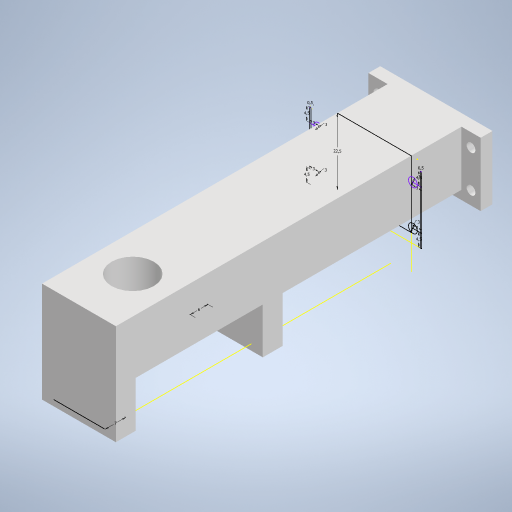
# Autodesk Inventor part: ramie_1
Saved by Autodesk Inventor 2023 (Build 270158000, 158)
## iProperties
Created: 2022-09-14
Part Number: ramie_1
Material: Generic
Document SubType Name: Modeling
Designer: Kamil
Density: 1 g/cm^3
Appearance: Default
Author: Kamil
Autodesk Inventor part; units mm, degrees
ref_plane "YZ Plane" through (0, 0, 0) normal (1, 0, 0) x (0, 1, 0)
ref_plane "XZ Plane" through (0, 0, 0) normal (0, 1, 0) x (-1, 0, 0)
ref_plane "XY Plane" through (0, 0, 0) normal (0, 0, 1) x (1, 0, 0)
sketch "Sketch14" plane through (0, 0, 0) normal (0, 0, 1) x (1, 0, 0)
  line L0 (0, 0) -> (17, 0)
  line L1 (17, 0) -> (17, 30)
  line L2 (17, 30) -> (0, 30)
  line L3 (0, 30) -> (0, 0)
  line L4 (-6, 36) -> (23, 36)
  line L5 (23, 36) -> (23, -6)
  line L6 (23, -6) -> (-6, -6)
  line L7 (-6, -6) -> (-6, 36)
  dimension "d55" = 17
  dimension "d56" = 30
  dimension "d57" = 6
  constraints: 16 end point, 4 parallel, 2 perpendicular, 1 horizontal, 3 other
  measures "d55" distance of L2.end L1.end
  measures "d56" distance of L1.end L0.end
  measures "d57" distance between parallel lines of L2 L4
extrude "Extrusion12" add sketch "Sketch14" against normal blind 3 contours L3 L2 L1 L0 | L4 L5 L6 L7
extrude "Extrusion13" add sketch "Sketch14" along normal blind 90 contours L3 L2 L1 L0
sketch "Sketch15" plane through (0, 0, 0) normal (0, -1, 0) x (1, 0, 0)
  line L0 (0, 0) -> (0, 90) projected
  line L1 (0, 90) -> (17.1111, 90)
  line L2 (0, 90) -> (17, 90)
  line L3 (17, 90) -> (17, 97)
  line L4 (17, 97) -> (0, 97)
  line L5 (0, 97) -> (0, 90)
  line L6 (17, 90) -> (0, 90) projected
  circle A0 centre (3.5, 93.5) radius 1.25
  circle A1 centre (13.5, 93.5) radius 1.25
  line L7 (8.5, 113.1) -> (8.5, 78.8)
  circle A2 centre (8.5, 78.8) radius 7.15
  circle A3 centre (3.5, 44) radius 1.25
  circle A4 centre (13.5, 44) radius 1.25
  line L8 (17, 0) -> (17, 90) projected
  line L9 (0, 97) -> (17, 97)
  line L10 (17, 97) -> (17, 42)
  line L11 (17, 42) -> (0, 42)
  line L12 (0, 42) -> (0, 97)
  line L13 (8.5, 113.1) -> (8.5, 98.4)
  line L14 (3.5, 44) -> (13.5, 44)
  dimension "d67" = 7
  dimension "d70" = 2.5
  dimension "d71" = 2.5
  dimension "d72" = 34.3
  dimension "d73" = 14.3
  dimension "d79" = 55
  dimension "d95" = 14.7
  constraints: 24 end point, 5 centre point, 4 parallel, 3 horizontal, 2 perpendicular, 2 point on line, 1 coincident, 1 vertical
  measures "d67" distance of L3.end L2.end
  measures "d70" diameter of A0
  measures "d71" diameter of A1
  measures "d72" distance of L7.start L7.end
  measures "d73" diameter of A2
  measures "d79" distance of L9.end L10.end
  measures "d95" distance of L7.start L13.end
extrude "Extrusion14" cut sketch "Sketch15" against normal blind 169.375 contours A2
extrude "Extrusion15" cut sketch "Sketch15" against normal blind 15.5 contours L0 L1 L8 L11
extrude "Extrusion16" cut sketch "Sketch15" against normal blind 20 contours A3 | A4
extrude "Extrusion17" add sketch "Sketch15" against normal blind 30 contours L5 L4 L7 L1 | L7 L4 L3 L1
sketch "Sketch16" plane through (0, 0, 0) normal (0, -1, 0) x (1, 0, 0)
  line L0 (0, 0) -> (0, 97) projected
  line L1 (17, 0) -> (17, 97) projected
  line L2 (0, 97) -> (17, 97)
  line L3 (17, 97) -> (17, 90)
  line L4 (17, 90) -> (0, 90)
  line L5 (0, 90) -> (0, 97)
  dimension "d86" = 7
  constraints: 8 end point, 2 parallel, 1 horizontal, 1 perpendicular, 1 point on line
  measures "d86" distance of L2.end L3.end
extrude "Extrusion18" cut sketch "Sketch15" against normal blind 15.5 contours L5 L4 L7 L1 | L7 L4 L3 L1
sketch "Sketch17" plane through (0, 15.5, 0) normal (0, -1, 0) x (1, 0, 0)
  line L0 (0, 97) -> (17, 97) projected
  line L1 (17, 0) -> (17, 97) projected
  line L2 (0, 97) -> (17, 97)
  line L3 (17, 97) -> (17, 91)
  line L4 (17, 91) -> (0, 91)
  line L5 (0, 91) -> (0, 97)
  line L6 (17, 42) -> (0, 42) projected
  line L7 (0, 42) -> (17, 42)
  line L8 (17, 42) -> (17, 47)
  line L9 (17, 47) -> (0, 47)
  line L10 (0, 47) -> (0, 42)
  circle A0 centre (3.5, 44) radius 1.25 projected
  circle A1 centre (3.5, 44) radius 1.25
  circle A2 centre (13.5, 44) radius 1.25 projected
  circle A3 centre (13.5, 44) radius 1.25
  circle A4 centre (3.5, 93.5) radius 1.25 projected
  circle A5 centre (3.5, 93.5) radius 1.25
  circle A6 centre (13.5, 93.5) radius 1.25 projected
  circle A7 centre (13.5, 93.5) radius 1.25
  point P0 (0, 0)
  dimension "d89" = 6
  dimension "d90" = 5
  dimension "d91" = 2.5
  dimension "d92" = 2.5
  constraints: 16 end point, 4 centre point, 4 coincident, 4 parallel, 2 horizontal, 2 perpendicular, 2 point on line
  measures "d89" distance of L2.end L3.end
  measures "d90" distance of L8.end L7.end
  measures "d91" diameter of A5
  measures "d92" diameter of A7
extrude "Extrusion19" add sketch "Sketch17" along normal blind 15.5
sketch "Sketch19" plane through (0, 0, 0) normal (0, -1, 0) x (1, 0, 0)
  line L0 (0, 0) -> (0, 47) projected
  line L1 (17, 0) -> (17, 47) projected
  line L2 (0, 0) -> (17, 0)
  line L3 (17, 0) -> (17, 40)
  line L4 (17, 40) -> (0, 40)
  line L5 (0, 40) -> (0, 0)
  dimension "d96" = 40
  constraints: 8 end point, 2 parallel, 1 horizontal, 1 perpendicular, 1 point on line
  measures "d96" distance of L3.end L2.end
extrude "Extrusion20" cut sketch "Sketch19" against normal blind 15.5
sketch "Sketch23" plane through (0, 0, 0) normal (0, 0, 1) x (1, 0, 0)
  line L0 (0, 15.5) -> (17, 15.5) projected
  line L1 (0, 15.5) -> (0, 9.5)
  line L2 (0, 15.5) -> (0, 0) projected
  line L3 (0, 9.5) -> (-6, 9.5)
  line L4 (-6, -6) -> (-6, 36) projected
  line L5 (23, 36) -> (23, -6) projected
  line L6 (23, 9.5) -> (0, 9.5)
  line L7 (-6, 9.5) -> (23, 9.5)
  line L8 (23, 9.5) -> (23, 36)
  line L9 (23, 36) -> (-6, 36)
  line L10 (-6, 36) -> (-6, 9.5)
  line L11 (23, -6) -> (-6, -6) projected
  line L12 (-6, -6) -> (23, -6)
  line L13 (23, -6) -> (23, 9.5)
  line L14 (23, 9.5) -> (-6, 9.5)
  line L15 (-6, 9.5) -> (-6, -6)
  dimension "d99" = 6
  constraints: 22 end point, 4 parallel, 4 perpendicular, 4 point on line, 2 horizontal
  measures "d99" distance of L0.start L1.end
extrude "Extrusion21" cut sketch "Sketch23" against normal blind 15.5 contours L6 L5 L11 L4 L3
sketch "Sketch24" plane through (0, 30, 97) normal (0, 0, 1) x (1, 0, 0)
  line L0 (17, 0) -> (17, -14.5) projected
  line L1 (17, 0) -> (19, 0)
  line L2 (19, 0) -> (19, 2)
  line L3 (0, -14.5) -> (0, -30) projected
  line L4 (0, -14.5) -> (-2, -14.5)
  line L5 (-2, -14.5) -> (-2, -16.5)
  line L6 (-2, -16.5) -> (19, -16.5)
  line L7 (19, -16.5) -> (19, 2)
  line L8 (19, 2) -> (-2, 2)
  line L9 (-2, 2) -> (-2, -16.5)
  dimension "d111" = 2
  dimension "d112" = 2
  dimension "d113" = 2
  dimension "d114" = 2
  constraints: 16 end point, 3 horizontal, 3 perpendicular, 2 parallel
  measures "d111" distance of L0.start L1.end
  measures "d112" distance of L1.end L2.end
  measures "d113" distance of L3.start L4.end
  measures "d114" distance of L4.end L5.end
extrude "Extrusion22" add sketch "Sketch24" against normal blind 97
extrude "Extrusion23" cut sketch "Sketch15" against normal blind 169.375 contours A2
sketch "Sketch26" plane through (-2, 13.5, 0) normal (0, -1, 0) x (1, 0, 0)
  line L0 (0, 97) -> (2, 97) projected
  line L1 (2, 97) -> (2, 91) projected
  line L2 (0, 97) -> (2, 97)
  line L3 (2, 97) -> (2, 91)
  line L4 (2, 91) -> (0, 91)
  line L5 (0, 91) -> (0, 97)
  line L6 (2, 91) -> (19, 91) projected
  line L7 (19, 97) -> (21, 97) projected
  line L8 (19, 91) -> (21, 91)
  line L9 (21, 91) -> (21, 97)
  line L10 (21, 97) -> (19, 97)
  line L11 (19, 97) -> (19, 91)
  line L12 (2, 40) -> (19, 40) projected
  line L13 (0, 97) -> (0, 0) projected
  line L14 (2, 40) -> (0, 40)
  line L15 (0, 40) -> (0, 47)
  line L16 (0, 47) -> (2, 47)
  line L17 (2, 47) -> (2, 40)
  line L18 (19, 40) -> (19, 47) projected
  line L19 (21, 97) -> (21, 0) projected
  line L20 (19, 40) -> (21, 40)
  line L21 (21, 40) -> (21, 47)
  line L22 (21, 47) -> (19, 47)
  line L23 (19, 47) -> (19, 40)
  point P0 (2, 0)
  point P1 (0, 40)
  dimension "d119" = 7
  constraints: 32 end point, 8 parallel, 4 horizontal, 4 perpendicular, 3 point on line
  measures "d119" distance of L14.end L15.end
extrude "Extrusion24" add sketch "Sketch26" along normal blind 13.5 contours L0 L1 L4 L5 | L16 L17 L14 L13 | L11 L7 L9 L8 | L19 L20 L18 L22
sketch "Sketch27" plane through (0, 0, 0) normal (0, 0, 1) x (1, 0, 0)
  point P0 (0, 0)
sketch "Sketch28" plane through (0, 0, 0) normal (0, 0, 1) x (1, 0, 0)
  line L0 (-6, 9.5) -> (-6, 36) projected
  line L1 (-6, 36) -> (23, 36) projected
  line L2 (-6, 31.9237) -> (23, 31.9237)
  line L3 (23, 31.9237) -> (23, 36)
  line L4 (23, 36) -> (-6, 36)
  line L5 (-6, 36) -> (-6, 31.9237)
  point P0 (0, 0)
  constraints: 8 end point, 2 parallel, 1 horizontal, 1 perpendicular, 1 point on line
extrude "Extrusion25" cut sketch "Sketch28" against normal blind 13.5
sketch "Sketch29" plane through (0, 0, 0) normal (0, -1, 0) x (1, 0, 0)
  point P0 (0, 0)
sketch "Sketch30" plane through (0, 0, 0) normal (0, -1, 0) x (1, 0, 0)
  line L0 (19, 97) -> (-2, 97) projected
  line L1 (-2, 91) -> (19, 91) projected
  line L2 (-2, 97) -> (19, 97)
  line L3 (19, 97) -> (19, 91)
  line L4 (19, 91) -> (-2, 91)
  line L5 (-2, 91) -> (-2, 97)
  line L6 (-2, 47) -> (-2, 40) projected
  line L7 (-2, 40) -> (19, 40) projected
  line L8 (-2, 47) -> (19, 47)
  line L9 (19, 47) -> (19, 40)
  line L10 (19, 40) -> (-2, 40)
  line L11 (-2, 40) -> (-2, 47)
  circle A0 centre (3.5, 93.5) radius 1.25 projected
  circle A1 centre (3.5, 93.5) radius 1.25
  circle A2 centre (13.5, 93.5) radius 1.25 projected
  circle A3 centre (13.5, 93.5) radius 1.25
  circle A4 centre (3.5, 44) radius 1.25 projected
  circle A5 centre (3.5, 44) radius 1.25
  circle A6 centre (13.5, 44) radius 1.25 projected
  circle A7 centre (13.5, 44) radius 1.25
  point P0 (0, 0)
  constraints: 16 end point, 4 centre point, 4 coincident, 4 parallel, 2 horizontal, 2 perpendicular
extrude "Extrusion26" add sketch "Sketch30" along normal blind 2
sketch "Sketch31" plane through (0, 0, -3) normal (0, 0, -1) x (-1, 0, 0)
  point P0 (0, 0)
  point P1 (6, 9.5)
  point P2 (-23, 31.9237)
sketch "Sketch32" plane through (-2, 13.5, 47) normal (0, -1, 0) x (1, 0, 0)
  point P0 (2, -47)
sketch "Sketch33" plane through (-2, 32, 97) normal (0, 0, 1) x (1, 0, 0)
  line L0 (21, -34) -> (21, 0) projected
  line L1 (-4, -22.5) -> (25, -22.5) projected
  line L2 (21, 0) -> (23, 0)
  line L3 (23, 0) -> (23, -22.5)
  line L4 (23, -22.5) -> (21, -22.5)
  line L5 (21, -22.5) -> (21, 0)
  line L6 (0, -18.5) -> (0, -34) projected
  line L7 (-4, -0.0763) -> (25, -0.0763) projected
  line L8 (0, -22.5) -> (-2, -22.5)
  line L9 (-2, -22.5) -> (-2, -0.0763)
  line L10 (-2, -0.0763) -> (0, -0.0763)
  line L11 (0, -0.0763) -> (0, -22.5)
  line L12 (0, -18.5) -> (-2, -18.5)
  line L13 (21, -18.5) -> (21, -34) projected
  line L14 (21, -18.5) -> (23, -18.5)
  point P0 (2, -32)
  point P1 (0, -0.0763)
  point P2 (23, -0.0763)
  point P3 (21, -0.0763)
  dimension "d126" = 2
  dimension "d127" = 2
  constraints: 20 end point, 6 point on line, 4 parallel, 4 perpendicular, 2 horizontal
  measures "d126" distance of L3.end L4.end
  measures "d127" distance of L9.end L10.end
extrude "Extrusion27" add sketch "Sketch33" against normal blind 100 contours L0 L7 L3 L14 | L12 L9 L7 L11
sketch "Sketch34" plane through (0, -2, 0) normal (0, -1, 0) x (1, 0, 0)
  line L0 (-2, 47) -> (19, 47) projected
  line L1 (-2, 47) -> (-2, 40) projected
  line L2 (19, 47) -> (-2, 47)
  line L3 (-2, 47) -> (-2, 41)
  line L4 (-2, 41) -> (19, 41)
  line L5 (19, 41) -> (19, 47)
  line L6 (-2, 40) -> (19, 40) projected
  line L7 (19, 41) -> (-2, 41)
  line L8 (-2, 41) -> (-2, 40)
  line L9 (-2, 40) -> (19, 40)
  line L10 (19, 40) -> (19, 41)
  point P0 (0, 0)
  dimension "d130" = 6
  constraints: 16 end point, 4 parallel, 2 horizontal, 2 perpendicular, 1 point on line
  measures "d130" distance of L3.end L2.end
sketch "Sketch35" plane through (0, -2, 0) normal (0, -1, 0) x (1, 0, 0)
  line L0 (-2, 47) -> (19, 47) projected
  line L1 (-2, 47) -> (-2, 91) projected
  line L2 (19, 47) -> (-2, 47)
  line L3 (-2, 47) -> (-2, 46.5)
  line L4 (-2, 46.5) -> (19, 46.5)
  line L5 (19, 46.5) -> (19, 47)
  line L6 (-2, 40) -> (19, 40) projected
  line L7 (-2, 47) -> (-2, 40) projected
  line L8 (19, 40) -> (-2, 40)
  line L9 (-2, 40) -> (-2, 40.5)
  line L10 (-2, 40.5) -> (19, 40.5)
  line L11 (19, 40.5) -> (19, 40)
  point P0 (0, 0)
  point P1 (-2, 41)
  dimension "d133" = 0.5
  dimension "d136" = 0.5
  constraints: 16 end point, 4 parallel, 2 horizontal, 2 perpendicular, 2 point on line
  measures "d133" distance of L3.end L2.end
  measures "d136" distance of L8.end L9.end
extrude "Extrusion29" cut sketch "Sketch35" against normal blind 15.5 contours L0 L5 L4 L3
extrude "Extrusion30" cut sketch "Sketch35" against normal blind 15.5 contours L10 L11 L6 L7
sketch "Sketch36" plane through (-2, 13.5, 91) normal (0, -1, 0) x (1, 0, 0)
  line L0 (-2, 6) -> (0, 6) projected
  line L1 (21, 0) -> (0, 0) projected
  line L2 (-2, 6) -> (0, 6)
  line L3 (0, 6) -> (0, 0)
  line L4 (0, 0) -> (-2, 0)
  line L5 (-2, 0) -> (-2, 6)
  line L6 (21, 0) -> (21, 6) projected
  line L7 (23, 6) -> (23, -91) projected
  line L8 (21, 6) -> (23, 6)
  line L9 (23, 6) -> (23, 0)
  line L10 (23, 0) -> (21, 0)
  line L11 (21, 0) -> (21, 6)
  line L12 (21, -44.5) -> (0, -44.5) projected
  line L13 (-2, 6) -> (-2, -91) projected
  line L14 (0, -44.5) -> (-2, -44.5)
  line L15 (-2, -44.5) -> (-2, -50.5)
  line L16 (-2, -50.5) -> (0, -50.5)
  line L17 (0, -50.5) -> (0, -44.5)
  line L18 (21, -44.5) -> (23, -44.5)
  line L19 (23, -44.5) -> (23, -50.5)
  line L20 (23, -50.5) -> (21, -50.5)
  line L21 (21, -50.5) -> (21, -44.5)
  point P0 (2, -91)
  point P1 (23, -44.5)
  dimension "d139" = 6
  constraints: 32 end point, 8 parallel, 5 point on line, 4 horizontal, 4 perpendicular
  measures "d139" distance of L15.end L14.end
extrude "Extrusion31" add sketch "Sketch36" along normal blind 15.5 contours L0 L3 L4 L5 | L14 L17 L16 L13 | L6 L8 L7 L10 | L18 L7 L20 L21
sketch "Sketch37" plane through (0, 0, -3) normal (0, 0, -1) x (-1, 0, 0)
  line L0 (-23, 9.5) -> (6, 9.5) projected
  line L1 (-23, 9.5) -> (6, 9.5)
  line L2 (6, 9.5) -> (6, 32)
  line L3 (6, 32) -> (-23, 32)
  line L4 (-23, 32) -> (-23, 9.5)
  point P0 (0, 0)
  point P1 (6, 9.5)
  dimension "d142" = 29
  constraints: 8 end point, 2 parallel, 1 horizontal, 1 perpendicular
  measures "d142" distance of L3.end L2.end
extrude "Extrusion32" add sketch "Sketch37" against normal blind 3
sketch "Sketch38" plane through (0, 0, -3) normal (0, 0, -1) x (-1, 0, 0)
  line L0 (-23, 9.5) -> (6, 9.5) projected
  line L1 (-23, 9.5) -> (-27, 9.5)
  line L2 (-27, 9.5) -> (-27, 32)
  line L3 (6, 32) -> (-23, 32) projected
  line L4 (-27, 32) -> (6, 32)
  line L5 (6, 9.5) -> (10, 9.5)
  line L6 (10, 9.5) -> (10, 32)
  line L7 (10, 32) -> (-27, 32)
  point P0 (0, 0)
  dimension "d145" = 4
  dimension "d146" = 4
  constraints: 12 end point, 3 perpendicular, 2 horizontal, 1 collinear
  measures "d145" distance of L0.start L1.end
  measures "d146" distance of L0.end L5.end
extrude "Extrusion33" add sketch "Sketch38" against normal blind 3
sketch "Sketch39" plane through (0, 0, 0) normal (0, 0, 1) x (1, 0, 0)
  line L0 (21, 31.9237) -> (19, 31.9237) projected
  line L1 (19, 32) -> (19, 31.9237) projected
  line L2 (21, 31.9237) -> (19, 31.9237)
  line L3 (19, 31.9237) -> (19, 32)
  line L4 (19, 32) -> (21, 32)
  line L5 (21, 32) -> (21, 31.9237)
  line L6 (-2, 31.9237) -> (-2, 32) projected
  line L7 (-2, 31.9237) -> (-4, 31.9237) projected
  line L8 (-2, 32) -> (-4, 32)
  line L9 (-4, 32) -> (-4, 31.9237)
  line L10 (-4, 31.9237) -> (-2, 31.9237)
  line L11 (-2, 31.9237) -> (-2, 32)
  point P0 (0, 0)
  constraints: 16 end point, 4 parallel, 2 horizontal, 2 perpendicular
extrude "Extrusion34" add sketch "Sketch39" along normal blind 97
sketch "Sketch40" plane through (0, 0, 0) normal (0, 0, 1) x (1, 0, 0)
  point P0 (0, 0)
sketch "Sketch41" plane through (0, 0, 0) normal (0, 0, 1) x (1, 0, 0)
  line L0 (-10, 32) -> (-10, 27.5)
  line L1 (-10, 32) -> (-10, 9.5) projected
  line L2 (-10, 9.5) -> (27, 9.5) projected
  line L3 (-10, 9.5) -> (-10, 14)
  line L4 (-10, 9.5) -> (-10.5, 9.5)
  line L5 (-10.5, 9.5) -> (-10.5, 32)
  line L6 (-10.5, 32) -> (-10, 32)
  line L7 (-10, 32) -> (-10, 9.5)
  line L8 (-10.5, 14) -> (-7.5, 14)
  line L9 (-10.5, 27.5) -> (-7.5, 27.5)
  circle A0 centre (-7.5, 14) radius 1.5
  circle A1 centre (-7.5, 27.5) radius 1.5
  line L10 (27, 9.5) -> (27, 32) projected
  line L11 (27, 9.5) -> (27.5, 9.5)
  line L12 (27.5, 9.5) -> (27.5, 32)
  line L13 (27.5, 32) -> (27, 32)
  line L14 (27, 32) -> (27, 9.5)
  line L15 (27.5, 9.5) -> (27.5, 14)
  line L16 (27.5, 14) -> (24.5, 14)
  line L17 (27.5, 32) -> (27.5, 27.5)
  line L18 (27.5, 27.5) -> (24.5, 27.5)
  circle A2 centre (24.5, 14) radius 1.5
  circle A3 centre (24.5, 27.5) radius 1.5
  point P0 (0, 0)
  dimension "d151" = 4.5
  dimension "d152" = 4.5
  dimension "d153" = 0.5
  dimension "d154" = 3
  dimension "d155" = 3
  dimension "d156" = 3
  dimension "d157" = 3
  dimension "d158" = 0.5
  dimension "d159" = 4.5
  dimension "d160" = 3
  dimension "d161" = 4.5
  dimension "d162" = 3
  dimension "d163" = 3
  dimension "d164" = 3
  constraints: 32 end point, 6 point on line, 5 perpendicular, 4 centre point, 4 coincident, 4 parallel, 3 horizontal
  measures "d151" distance of L0.start L0.end
  measures "d152" distance of L1.end L3.end
  measures "d153" distance of L5.end L6.end
  measures "d154" distance of L8.start L8.end
  measures "d155" distance of L9.start L9.end
  measures "d156" diameter of A0
  measures "d157" diameter of A1
  measures "d158" distance of L13.end L12.end
  measures "d159" distance of L11.end L15.end
  measures "d160" distance of L15.end L16.end
  measures "d161" distance of L12.end L17.end
  measures "d162" distance of L17.end L18.end
  measures "d163" diameter of A2
  measures "d164" diameter of A3
sketch "Sketch42" plane through (0, 0, -3) normal (0, 0, -1) x (-1, 0, 0)
  point P0 (0, 0)
sketch "Sketch43" plane through (0, 0, -3) normal (0, 0, -1) x (-1, 0, 0)
  line L0 (-21, -2) -> (-21, 32) projected
  line L1 (4, 13.5) -> (4, -2) projected
  line L2 (-21, 32) -> (4, 32)
  line L3 (4, 32) -> (4, 9.5)
  line L4 (4, 9.5) -> (-21, 9.5)
  line L5 (-21, 9.5) -> (-21, 32)
  point P0 (0, 0)
  dimension "d165" = 22.5
  constraints: 8 end point, 2 parallel, 1 horizontal, 1 perpendicular, 1 point on line
  measures "d165" distance of L2.end L3.end
sketch "Sketch44" plane through (0, 0, -3) normal (0, 0, -1) x (-1, 0, 0)
  line L0 (10, 9.5) -> (10, 32) projected
  line L1 (10, 9.5) -> (-28.3786, 9.5)
  line L2 (-28.3786, 9.5) -> (-28.3786, 33.0505)
  line L3 (-28.3786, 33.0505) -> (10, 33.0505)
  line L4 (10, 33.0505) -> (10, 9.5)
  point P0 (0, 0)
  constraints: 8 end point, 2 parallel, 1 horizontal, 1 perpendicular
extrude "Extrusion35" cut sketch "Sketch44" against normal blind 3
sketch "Sketch45" plane through (0, 0, 0) normal (0, 0, -1) x (-1, 0, 0)
  line L0 (4, 13.5) -> (-21, 13.5) projected
  line L1 (4, 32) -> (4, -2) projected
  line L2 (-21, 13.5) -> (4, 13.5)
  line L3 (4, 13.5) -> (4, 32)
  line L4 (4, 32) -> (-21, 32)
  line L5 (-21, 32) -> (-21, 13.5)
  point P0 (0, 0)
  constraints: 8 end point, 2 parallel, 1 horizontal, 1 perpendicular
extrude "Extrusion36" add sketch "Sketch45" along normal blind 20
sketch "Sketch46" plane through (0, 0, -20) normal (0, 0, -1) x (-1, 0, 0)
  line L0 (-21, 32) -> (4, 32) projected
  line L1 (-21, 32) -> (-27.5, 32)
  line L2 (-27.5, 32) -> (-27.5, 13.5)
  line L3 (-27.5, 13.5) -> (-21, 13.5)
  line L4 (-21, 13.5) -> (-21, 32)
  line L5 (4, 32) -> (4, -2) projected
  line L6 (4, 32) -> (10.5, 32)
  line L7 (10.5, 32) -> (10.5, 13.5)
  line L8 (10.5, 13.5) -> (4, 13.5)
  line L9 (4, 13.5) -> (4, 32)
  line L10 (10.5, 13.5) -> (-27.5, 13.5)
  point P0 (0, 0)
  constraints: 18 end point, 4 parallel, 3 horizontal, 2 perpendicular
extrude "Extrusion37" add sketch "Sketch46" along normal blind 4
sketch "Sketch47" plane through (0, 0, -20) normal (0, 0, 1) x (1, 0, 0)
  line L0 (-4, 13.5) -> (-10.5, 13.5) projected
  line L1 (-10.5, 13.5) -> (27.5, 13.5)
  line L2 (27.5, 13.5) -> (27.5, 10.5)
  line L3 (27.5, 10.5) -> (-10.5, 10.5)
  line L4 (-10.5, 10.5) -> (-10.5, 13.5)
  point P0 (0, 0)
  dimension "d175" = 3
  constraints: 8 end point, 2 parallel, 1 horizontal, 1 perpendicular
  measures "d175" distance of L1.end L2.end
extrude "Extrusion38" add sketch "Sketch47" against normal blind 4
sketch "Sketch48" plane through (0, 0, -20) normal (0, 0, 1) x (1, 0, 0)
  line L0 (-10.5, 10.5) -> (27.5, 10.5) projected
  line L1 (-10.5, 10.5) -> (-10.5, 15)
  line L2 (-10.5, 10.5) -> (-10.5, 32) projected
  line L3 (-10.5, 15) -> (-7.25, 15)
  line L4 (-10.5, 32) -> (-10.5, 27.5)
  line L5 (-10.5, 27.5) -> (-7.25, 27.5)
  circle A0 centre (-7.25, 15) radius 1.5
  circle A1 centre (-7.25, 27.5) radius 1.5
  line L6 (27.5, 32) -> (27.5, 10.5) projected
  line L7 (27.5, 10.5) -> (27.5, 15)
  line L8 (27.5, 15) -> (27.5, 18)
  line L9 (27.5, 15) -> (24.25, 15)
  line L10 (-10.5, 32) -> (27.5, 32) projected
  line L11 (27.5, 32) -> (27.5, 27.5)
  line L12 (27.5, 27.5) -> (24.25, 27.5)
  circle A2 centre (24.25, 27.5) radius 1.5
  circle A3 centre (24.25, 15) radius 1.5
  line L13 (-7.5, 15) -> (-7.25, 15)
  line L14 (24.5, 15) -> (24.25, 15)
  point P0 (0, 0)
  dimension "d178" = 4.5
  dimension "d180" = 4.5
  dimension "d184" = 4.5
  dimension "d185" = 3
  dimension "d187" = 4.5
  dimension "d195" = 0.25
  constraints: 22 end point, 5 point on line, 4 centre point, 4 coincident, 3 horizontal, 3 perpendicular
  measures "d178" distance of L0.start L1.end
  measures "d180" distance of L2.end L4.end
  measures "d184" distance of L0.end L7.end
  measures "d185" distance of L7.end L8.end
  measures "d187" distance of L6.start L11.end
  measures "d195" distance of L14.start L14.end
extrude "Extrusion39" cut sketch "Sketch48" against normal blind 4 contours A3 | A2 | A1 | A0
sketch "Sketch49" plane through (0, -2, 0) normal (0, -1, 0) x (1, 0, 0)
  point P0 (0, 0)
sketch "Sketch50" plane through (-4, 13.5, 91) normal (0, -1, 0) x (1, 0, 0)
  point P0 (4, -91)
sketch "019855" plane through (-4, 13.5, 91) normal (0, -1, 0) x (1, 0, 0)
  circle A0 centre (12.5, -12.2) radius 7.15 projected
  line L0 (19.65, -10.7) -> (19.65, -13.7)
  line L1 (19.65, -13.7) -> (19.65, -12.2)
  line L2 (5.35, -10.7) -> (5.35, -13.7)
  line L3 (5.5091, -12.2) -> (5.35, -12.2)
  line L4 (19.65, -10.7) -> (19.65, -13.7)
  line L5 (5.35, -13.7) -> (5.35, -10.7)
  point P0 (4, -91)
  point P1 (19.65, -12.2)
  constraints: 12 end point, 1 horizontal, 1 parallel, 1 tangent
thread "Thread5" size "M2.5x0.45" class "6H" standard "ANSI Metric M Profile" full length
thread "Thread6" size "M2.5x0.45" class "6H" standard "ANSI Metric M Profile" full length
thread "Thread7" size "M2.5x0.45" class "6H" standard "ANSI Metric M Profile" full length
thread "Thread8" size "M2.5x0.45" class "6H" standard "ANSI Metric M Profile" full length
sketch "Sketch52" plane through (0, -2, 0) normal (0, -1, 0) x (1, 0, 0)
  point P0 (0, 0)
sketch "Sketch53" plane through (-4, 13.5, 91) normal (0, -1, 0) x (1, 0, 0)
  line L0 (0, 0) -> (25, 0) projected
  line L1 (25, 6) -> (25, -111) projected
  line L2 (0, 0) -> (25, 0)
  line L3 (25, 0) -> (25, -0.5)
  line L4 (25, -0.5) -> (0, -0.5)
  line L5 (0, -0.5) -> (0, 0)
  line L6 (25, -44.5) -> (0, -44.5) projected
  line L7 (0, -44.5) -> (25, -44.5)
  line L8 (25, -44.5) -> (25, -44)
  line L9 (25, -44) -> (0, -44)
  line L10 (0, -44) -> (0, -44.5)
  line L11 (0, -44) -> (25, -44)
  line L12 (25, -44) -> (25, -43.75)
  line L13 (25, -43.75) -> (0, -43.75)
  line L14 (0, -43.75) -> (0, -44)
  line L15 (0, -0.5) -> (25, -0.5)
  line L16 (25, -0.5) -> (25, -0.75)
  line L17 (25, -0.75) -> (0, -0.75)
  line L18 (0, -0.75) -> (0, -0.5)
  point P0 (4, -91)
  dimension "d210" = 0.5
  dimension "d211" = 0.5
  dimension "d214" = 0.25
  dimension "d215" = 0.25
  constraints: 32 end point, 8 parallel, 4 horizontal, 4 perpendicular, 4 point on line
  measures "d210" distance of L2.end L3.end
  measures "d211" distance of L8.end L7.end
  measures "d214" distance of L12.end L11.end
  measures "d215" distance of L15.end L16.end
extrude "Extrusion42" add sketch "Sketch53" along normal blind 15.5 contours L0 L1 L4 L5 | L1 L6 L10 L9
extrude "Extrusion43" add sketch "Sketch53" along normal blind 15.5 contours L1 L9 L14 L13 | L4 L1 L17 L18
sketch "Sketch54" plane through (-4, 13.5, 90.25) normal (0, -1, 0) x (1, 0, 0)
  point P0 (4, -90.25)
sketch "Sketch55" plane through (-4, 13.5, 90.25) normal (0, -1, 0) x (1, 0, 0)
  point P0 (4, -90.25)
sketch "Sketch56" plane through (-4, 13.5, 90.25) normal (0, -1, 0) x (1, 0, 0)
  point P0 (4, -90.25)
body "Solid2"
